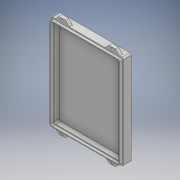
# Autodesk Inventor part: Top
Saved by Autodesk Inventor 2017 (Build 210142000, 142)
## iProperties
Created: 2017-05-28
Part Number: Top
Material: Generic
Document SubType Name: Modeling
Designer: William
Density: 1 g/cm^3
Appearance: Default
Author: William
Autodesk Inventor part; units mm, degrees
ref_plane "YZ Plane" through (0, 0, 0) normal (1, 0, 0) x (0, 1, 0)
ref_plane "XZ Plane" through (0, 0, 0) normal (0, 1, 0) x (-1, 0, 0)
ref_plane "XY Plane" through (0, 0, 0) normal (0, 0, 1) x (1, 0, 0)
sketch "Sketch1" plane through (0, 0, 0) normal (0, 1, 0) x (-1, 0, 0)
  circle A0 centre (-55, 111.5) radius 1.6
  circle A1 centre (-55.4645, -12) radius 1.6
  circle A2 centre (8, -12) radius 1.6
  circle A3 centre (8, 111.5) radius 1.6
  arc A4 (-67, 109) -> (-69, 107) centre (-67, 107) ccw
  line L0 (-69, 107) -> (-69, -7.5)
  arc A5 (-69, -7.5) -> (-67, -9.5) centre (-67, -7.5) ccw
  line L1 (-67, -9.5) -> (-64, -9.5)
  line L2 (-59, -14.5) -> (-64, -9.5)
  line L3 (-51, -14.5) -> (-59, -14.5)
  line L4 (-46, -9.5) -> (-51, -14.5)
  line L5 (-46, -9.5) -> (-1, -9.5)
  line L6 (-1, -9.5) -> (4, -14.5)
  line L7 (4, -14.5) -> (12, -14.5)
  line L8 (12, -14.5) -> (17, -9.5)
  line L9 (17, -9.5) -> (20, -9.5)
  arc A6 (20, -9.5) -> (22, -7.5) centre (20, -7.5) ccw
  line L10 (22, -7.5) -> (22, 107)
  arc A7 (22, 107) -> (20, 109) centre (20, 107) ccw
  line L11 (20, 109) -> (17, 109)
  line L12 (17, 109) -> (12, 114)
  line L13 (12, 114) -> (4, 114)
  line L14 (4, 114) -> (-1, 109)
  line L15 (-1, 109) -> (-46, 109)
  line L16 (-46, 109) -> (-51, 114)
  line L17 (-51, 114) -> (-59, 114)
  line L18 (-59, 114) -> (-64, 109)
  line L19 (-64, 109) -> (-67, 109)
  point P0 (0, 0)
  point P1 (0, 0)
  constraints: 40 end point, 8 centre point, 8 point on circle
extrude "Extrusion1" add sketch "Sketch1" along normal blind 10
sketch "Sketch4" plane through (0, 0, 0) normal (0, -1, 0) x (1, 0, 0)
  line L0 (65, 105) -> (-18, 105)
  line L1 (-18, 105) -> (-18, -5.5)
  line L2 (-18, -5.5) -> (65, -5.5)
  line L3 (65, -5.5) -> (65, 105)
  line L4 (1, 109) -> (46, 109) projected
  line L5 (46, -9.5) -> (1, -9.5) projected
  line L6 (-22, -7.5) -> (-22, 107) projected
  line L7 (69, 107) -> (69, -7.5) projected
  point P0 (0, 0)
  dimension "d2" = 4
  dimension "d3" = 4
  dimension "d4" = 4
  dimension "d5" = 4
  constraints: 8 end point, 2 parallel, 1 horizontal, 1 perpendicular
  measures "d2" distance between parallel lines of L4 L0
  measures "d3" distance between parallel lines of L5 L2
  measures "d4" distance between parallel lines of L6 L1
  measures "d5" distance between parallel lines of L7 L3
extrude "Extrusion2" cut sketch "Sketch4" against normal blind 6
fillet "Fillet1" radius 2 4 edges at (65, 3, 105) (-18, 3, 105) (65, 3, -5.5) (-18, 3, -5.5)
sketch "Sketch5" plane through (0, 10, 0) normal (0, 1, 0) x (1, 0, 0)
  line L0 (64, -109) -> (67, -109) projected
  line L1 (-40.3504, -169.2964) -> (66.299, -169.2964)
  line L2 (66.299, -169.2964) -> (66.299, -109)
  line L3 (66.299, -109) -> (-40.3504, -109)
  line L4 (-40.3504, -109) -> (-40.3504, -169.2964)
  line L5 (-53.7547, 54.3444) -> (65.5201, 54.3444)
  line L6 (65.5201, 54.3444) -> (65.5201, 9.5)
  line L7 (65.5201, 9.5) -> (-53.7547, 9.5)
  line L8 (-53.7547, 9.5) -> (-53.7547, 54.3444)
  point P0 (0, 0)
  constraints: 16 end point, 4 parallel, 2 horizontal, 2 perpendicular, 1 point on line
extrude "Extrusion3" cut sketch "Sketch5" against normal blind 6
sketch "Sketch6" plane through (0, 0, 0) normal (0, -1, 0) x (1, 0, 0)
  line L0 (67.5, 107.5) -> (-20.5, 107.5)
  line L1 (-20.5, 107.5) -> (-20.5, -8)
  line L2 (-20.5, -8) -> (67.5, -8)
  line L3 (67.5, -8) -> (67.5, 107.5)
  line L4 (67, -9.5) -> (-20, -9.5) projected
  line L5 (-22, -7.5) -> (-22, 107) projected
  line L6 (69, 107) -> (69, -7.5) projected
  line L7 (-20, 109) -> (67, 109) projected
  line L8 (66.5, 106.5) -> (-19.5, 106.5)
  line L9 (-19.5, 106.5) -> (-19.5, -7)
  line L10 (-19.5, -7) -> (66.5, -7)
  line L11 (66.5, -7) -> (66.5, 106.5)
  point P0 (0, 0)
  dimension "d11" = 1.5
  dimension "d12" = 1.5
  dimension "d13" = 1.5
  dimension "d14" = 1.5
  dimension "d15" = 1
  dimension "d16" = 1
  dimension "d17" = 1
  dimension "d18" = 1
  constraints: 16 end point, 4 parallel, 2 horizontal, 2 perpendicular
  measures "d11" distance between parallel lines of L4 L2
  measures "d12" distance between parallel lines of L5 L1
  measures "d13" distance between parallel lines of L6 L3
  measures "d14" distance between parallel lines of L7 L0
  measures "d15" distance between parallel lines of L1 L9
  measures "d16" distance between parallel lines of L2 L10
  measures "d17" distance between parallel lines of L3 L11
  measures "d18" distance between parallel lines of L0 L8
extrude "Extrusion4" add sketch "Sketch6" along normal blind 3
fillet "Fillet2" radius 2 8 edges at (-20.5, -1.5, 107.5) (67.5, -1.5, 107.5) (66.5, -1.5, 106.5) (-19.5, -1.5, 106.5) (-20.5, -1.5, -8) (-19.5, -1.5, -7) (67.5, -1.5, -8) (66.5, -1.5, -7)
body "Solid1"
